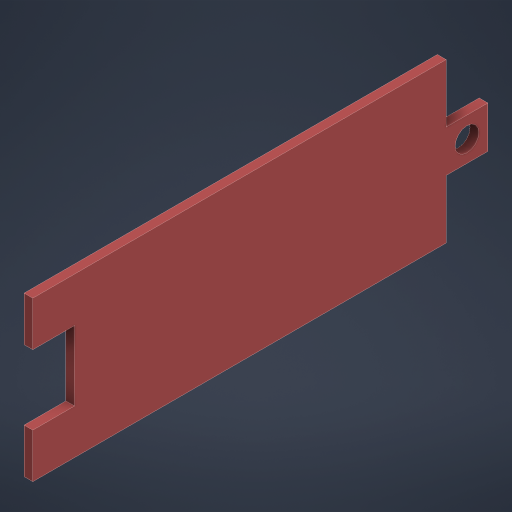
# Autodesk Inventor part: tapa_carcasa
Saved by Autodesk Inventor 2023.1 (Build 271208000, 208)
## iProperties
Created: 2022-11-07
Part Number: tapa_carcasa
Material: Generic
Document SubType Name: Modeling
Designer: amtat
Density: 1 g/cm^3
Appearance: Default
Author: amtat
Autodesk Inventor part; units mm, degrees
ref_plane "YZ Plane" through (0, 0, 0) normal (1, 0, 0) x (0, 1, 0)
ref_plane "XZ Plane" through (0, 0, 0) normal (0, 1, 0) x (-1, 0, 0)
ref_plane "XY Plane" through (0, 0, 0) normal (0, 0, 1) x (1, 0, 0)
sketch "Sketch1" plane through (0, 0, 0) normal (1, 0, 0) x (0, 1, 0)
  line L0 (0, 0) -> (0, -59.3)
  line L1 (0, -59.3) -> (22.8, -59.3)
  line L2 (22.8, -59.3) -> (22.8, 0)
  line L3 (22.8, 0) -> (0, 0)
  dimension "d0" = 59.3
  dimension "d1" = 22.8
  constraints: 8 end point, 2 perpendicular, 1 horizontal, 1 vertical
  measures "d0" distance of L0.start L0.end
  measures "d1" distance of L0.end L1.end
extrude "Extrusion1" add sketch "Sketch1" along normal blind 1.25
sketch "Sketch2" plane through (0, 0, 0) normal (0, 0, 1) x (1, 0, 0)
  line L0 (0, 22.8) -> (0, 0) projected
  line L1 (0, 0) -> (1.25, 0) projected
  line L2 (1.25, 22.8) -> (1.25, 0) projected
  line L3 (0, 22.8) -> (1.25, 22.8) projected
  line L4 (1.25, 0) -> (1.25, 22.8) projected
  line L5 (1.25, 22.8) -> (1.25, 11.4)
  line L6 (1.25, 11.4) -> (1.25, 16.4)
  line L7 (1.25, 16.4) -> (0, 16.4)
  line L8 (0, 0) -> (0, 22.8) projected
  line L9 (0, 16.4) -> (0, 6.4)
  line L10 (0, 6.4) -> (1.25, 6.4)
  dimension "d4" = 11.4
  dimension "d5" = 5
  dimension "d6" = 10
  constraints: 10 end point, 4 point on line, 2 perpendicular, 1 midpoint
  measures "d4" distance of L2.start L5.end
  measures "d5" distance of L5.end L6.end
  measures "d6" distance of L7.end L9.end
extrude "Extrusion2" cut sketch "Sketch2" against normal blind 6 contours L7 L2 L10 L0
sketch "Sketch3" plane through (1.25, 0, 0) normal (1, 0, 0) x (0, 0, -1)
  line L0 (6, 6.4) -> (0, 6.4) projected
  line L1 (0, 6.4) -> (0, 0) projected
  line L2 (0, 0) -> (59.3, 0) projected
  line L3 (59.3, 0) -> (59.3, 22.8) projected
  line L4 (59.3, 22.8) -> (0, 22.8) projected
  line L5 (0, 22.8) -> (0, 16.4) projected
  line L6 (0, 16.4) -> (6, 16.4) projected
  line L7 (6, 16.4) -> (6, 6.4) projected
  line L8 (59.3, 0) -> (59.3, 22.8) projected
  line L9 (59.3, 0) -> (59.3, 11.4)
  line L10 (59.3, 11.4) -> (59.3, 8.4)
  line L11 (59.3, 8.4) -> (65.3, 8.4)
  line L12 (65.3, 8.4) -> (65.3, 14.4)
  line L13 (65.3, 14.4) -> (59.3, 14.4)
  line L14 (59.3, 11.4) -> (62.3, 11.4)
  circle A0 centre (62.3, 11.4) radius 1.7
  dimension "d9" = 11.4
  dimension "d10" = 3
  dimension "d11" = 6
  dimension "d12" = 6
  dimension "d13" = 3.4
  constraints: 12 end point, 4 perpendicular, 2 point on line, 1 centre point, 1 coincident, 1 midpoint
  measures "d9" distance of L2.end L9.end
  measures "d10" distance of L9.end L10.end
  measures "d11" distance of L10.end L11.end
  measures "d12" distance of L11.end L12.end
  measures "d13" diameter of A0
extrude "Extrusion3" add sketch "Sketch3" against normal blind 1.25 contours L3 L13 L12 L11
body "Solid1"
